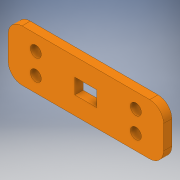
# Autodesk Inventor part: phone cord holder
Saved by Autodesk Inventor 2017 (Build 210142000, 142)
## iProperties
Created: 2018-11-02
Part Number: phone cord holder
Material: Generic
Document SubType Name: Modeling
Designer: Delta
Density: 1 g/cm^3
Appearance: Orange
Author: Delta
Autodesk Inventor part; units mm, degrees
ref_plane "YZ Plane" through (0, 0, 0) normal (1, 0, 0) x (0, 1, 0)
ref_plane "XZ Plane" through (0, 0, 0) normal (0, 1, 0) x (-1, 0, 0)
ref_plane "XY Plane" through (0, 0, 0) normal (0, 0, 1) x (1, 0, 0)
sketch "Sketch1" plane through (0, 0, 0) normal (0, 0, 1) x (1, 0, 0)
  line L0 (0, 0) -> (71.4502, 0)
  line L1 (71.4502, 0) -> (71.4502, -23.622)
  line L2 (71.4502, -23.622) -> (0, -23.622)
  line L3 (0, -23.622) -> (0, 0)
  dimension "d0" = 71.4502
  dimension "d1" = 23.622
  constraints: 8 end point, 2 parallel, 1 horizontal, 1 perpendicular
  measures "d0" distance of L1.end L2.end
  measures "d1" distance of L0.end L1.end
extrude "Extrusion1" add sketch "Sketch1" along normal blind 3.81
sketch "Sketch3" plane through (0, 0, 3.81) normal (0, 0, 1) x (1, 0, 0)
  line L0 (0, -23.622) -> (71.4502, -23.622) projected
  line L1 (71.4502, 0) -> (0, 0) projected
  line L2 (71.4502, -23.622) -> (71.4502, 0) projected
  point P0 (58.7248, -6.985)
  point P1 (58.7248, -16.637)
  dimension "d15" = 6.985
  dimension "d16" = 6.985
  dimension "d17" = 12.7254
  dimension "d18" = 12.7254
  measures "d15" distance from line of L0 point (58.725, -16.637)
  measures "d16" distance from line of L1 point (58.725, -6.985)
  measures "d17" distance from line of L2 point (58.725, -16.637)
  measures "d18" distance from line of L2 point (58.725, -6.985)
hole "Hole2" at (58.7248, -6.985, 3.81) at (58.7248, -16.637, 3.81) direction (0, 0, -1) diameter 5.08 depth 25.4 tip angle 118
ref_plane "Work Plane1" through (35.7251, -23.622, 0) normal (1, 0, 0) x (0, 0, -1)
mirror "Mirror1" about plane through (35.7251, -23.622, 0) normal (1, 0, 0) of "Hole2"
sketch "Sketch4" plane through (0, 0, 3.81) normal (0, 0, 1) x (1, 0, 0)
  line L0 (30.6451, -8.255) -> (40.8051, -8.255)
  line L1 (40.8051, -8.255) -> (40.8051, -15.367)
  line L2 (40.8051, -15.367) -> (30.6451, -15.367)
  line L3 (30.6451, -15.367) -> (30.6451, -8.255)
  line L4 (71.4502, -23.622) -> (71.4502, 0) projected
  line L5 (0, 0) -> (0, -23.622) projected
  line L6 (71.4502, 0) -> (0, 0) projected
  line L7 (0, -23.622) -> (71.4502, -23.622) projected
  dimension "d26" = 10.16
  dimension "d27" = 7.112
  dimension "d28" = 71.4502
  dimension "d29" = 30.6451
  dimension "d30" = 8.255
  dimension "d31" = 23.622
  constraints: 8 end point, 2 parallel, 1 horizontal, 1 perpendicular
  measures "d26" distance of L1.end L2.end
  measures "d27" distance of L0.end L1.end
  measures "d28" distance between parallel lines of L4 L5
  measures "d29" distance between parallel lines of L3 L5
  measures "d30" distance between parallel lines of L6 L0
  measures "d31" distance between parallel lines of L6 L7
extrude "Extrusion2" cut sketch "Sketch4" against normal blind 3.81 contours L0 L1 L2 L3
fillet "Fillet1" radius 6.35 4 edges at (71.4502, 0, 1.905) (71.4502, -23.622, 1.905) (0, 0, 1.905) (0, -23.622, 1.905)
equation "\"d16\" = d15"
equation "\"d17\" = d18"
body "Solid1"
